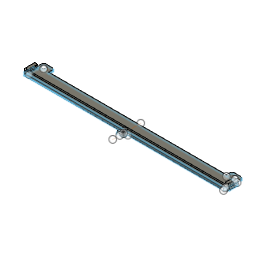
Light Bar v2 (Autodesk Fusion 360 design; units mm, degrees)
Autodesk Fusion 360 part; units mm, degrees
note: some values were not read from the file. Set by a fixed rule: which sketch regions a step uses.
sketch "base" plane through (0, 0, 0) normal (0, 1, 0) x (1, 0, 0)
  line L0 (-100, 1.5) -> (180, 1.5)
  line L1 (180, 1.5) -> (180, -13.5)
  line L2 (180, -13.5) -> (-100, -13.5)
  line L3 (-100, -13.5) -> (-100, 1.5)
  line L4 (-100, -13.5) -> (180, -13.5)
  line L5 (180, -13.5) -> (180, -17.5)
  line L6 (180, -17.5) -> (-100, -17.5)
  line L7 (-100, -17.5) -> (-100, -13.5)
  line L8 (-100, 1.5) -> (-85, 1.5) construction
  circle A0 centre (-94.5, 4) radius 2.5
  line L9 (-100, 1.5) -> (-100, 7.5)
  line L10 (-100, 7.5) -> (-98, 9.5)
  line L11 (-85, 1.5) -> (-85, 7.5)
  line L12 (-85, 7.5) -> (-87, 9.5)
  line L13 (-87, 9.5) -> (-98, 9.5)
  line L14 (40, 6.0385) -> (40, -33.3841) construction
  line L15 (167, 9.5) -> (178, 9.5)
  line L16 (180, 7.5) -> (178, 9.5)
  line L17 (180, 1.5) -> (180, 7.5)
  circle A1 centre (174.5, 4) radius 2.5
  line L18 (165, 7.5) -> (167, 9.5)
  line L19 (165, 1.5) -> (165, 7.5)
  circle A2 centre (40, -18.5) radius 2.5
  line L20 (34.5, -21.5) -> (36.5, -21.5) construction
  line L21 (36.5, -21.5) -> (36.5, -23.5) construction
  line L22 (34.5, -21.5) -> (36.5, -23.5)
  line L23 (36.5, -23.5) -> (40, -23.5)
  circle A3 centre (40, -18.5) radius 3.75 construction
  circle A4 centre (40, -18.5) radius 4
  line L24 (34.5, -21.5) -> (34.5, -17.5)
  line L25 (45.5, -21.5) -> (45.5, -17.5)
  line L26 (45.5, -21.5) -> (43.5, -23.5)
  line L27 (43.5, -23.5) -> (40, -23.5)
  line L28 (-98, -13) -> (-98, -1) construction
  line L29 (-98, -1) -> (-104, -1)
  line L30 (-104, -1) -> (-104, -13.5)
  line L31 (-104, -13.5) -> (-100, -17.5)
  line L32 (-98, -1) -> (-98, -13.5)
  line L33 (178, -13) -> (178, -1) construction
  line L34 (178, -1) -> (178, -13.5)
  line L35 (178, -1) -> (184, -1)
  line L36 (184, -1) -> (184, -13.5)
  line L37 (184, -13.5) -> (180, -17.5)
  circle A5 centre (-94.5, 4) radius 3.75 construction
  circle A6 centre (174.5, 4) radius 3.75 construction
  dimension "d1" = 280
  dimension "d2" = 15
  dimension "d3" = 4
  dimension "d4" = 280
  dimension "d5" = 15
  dimension "d7" = 5
  dimension "d8" = 2.5
  dimension "d11" = 140
  dimension "d16" = 5
  dimension "d17" = 5
  dimension "d20" = 2
  dimension "d21" = 2
  dimension "d22" = 7.5
  dimension "d23" = 8
  dimension "d29" = 12.5
  dimension "d42" = 7.5
  dimension "d43" = 7.5
  constraint horizontal L0
  constraint vertical L1
  constraint horizontal L2
  constraint vertical L3
  constraint horizontal L4
  constraint vertical L5
  constraint horizontal L6
  constraint vertical L7
  constraint horizontal L8
  constraint perpendicular L6 L14
  constraint symmetric L0.start L14 L0.end
  constraint symmetric L8.end L14 L19.start
  constraint symmetric A0 L14 A1
  constraint symmetric L9.end L14 L16.start
  constraint symmetric L10.end L14 L15.end
  constraint symmetric L11.end L14 L18.start
  constraint symmetric L12.end L14 L15.start
  constraint coincident L14 A2.centre
  constraint perpendicular L20 L21
  constraint coincident L14 L23.end
  constraint perpendicular L14 L23
  constraint concentric A2 A3
  constraint concentric A2 A4
  constraint coincident L6 L24.end
  constraint perpendicular L6 L24
  constraint symmetric L14 L20.start L25.start
  constraint symmetric L14 L21.end L26.end
  constraint symmetric L14 L23.end L27.end
  constraint symmetric L14 L24.end L25.end
  constraint parallel L3 L28
  constraint perpendicular L28 L29
  constraint perpendicular L29 L30
  constraint coincident L2 L32.end
  constraint perpendicular L2 L32
  constraint symmetric L6.end L14 L5.end
  constraint symmetric L14 L28.start L33.start
  constraint symmetric L14 L28.end L33.end
  constraint symmetric L14 L29.end L35.end
  constraint symmetric L14 L30.end L36.end
  constraint symmetric L14 L32.end L34.end
  constraint concentric A0 A5
  constraint concentric A1 A6
  measures "d1" distance of L0.start L0.end
  measures "d2" distance of L0.start L2.end
  measures "d3" distance of L2.end L6.end
  measures "d4" distance of L2.end L1.end
  measures "d5" distance of L0.start L8.end
  measures "d7" diameter of A0
  measures "d8" distance of L0 A0.centre
  measures "d11" distance of L3 L14
  measures "d16" diameter of A2
  measures "d17" distance of L4 A2.centre L0.start
  measures "d20" distance of L20.start L20.end L0.start
  measures "d21" distance of L20.end L21.end L0.start
  measures "d22" diameter of A3
  measures "d23" diameter of A4
  measures "d29" distance of L29.end L30.end
  measures "d42" diameter of A5
  measures "d43" diameter of A6
extrude "Extrude1" add sketch "base" along normal blind 2 contours L0 L1 L2 L3 L4 L29 L32 L34 L35 | L0 L9 L10 L11 L12 L13 | L0 L15 L16 L17 L18 L19 | L2 L3 L4 L29 L32 | L1 L2 L4 L34 L35 | L6 L22 L23 A4 L24 L25 L26 L27 | L6 A2 A4 | L6 A2 A4 makes body 1 at (-1.6667, 0, 8.5) makes body 2 at (39.9377, 0, 22.6643)
extrude "Extrude2" add sketch "base" along normal blind 5 contours L2 L4 L5 L6 L7 A4 bodies 1 2
chamfer "Chamfer1" distance 2 angle 45 2 edges at (-31.9365, 5, 17.5) (111.9365, 5, 17.5) on bodies 1
extrude "Extrude3" add sketch "base" along normal blind 6.5 contours L2 L3 L4 L29 L32 | L3 L7 L29 L30 L31 | L1 L5 L35 L36 L37 | L1 L2 L4 L34 L35 bodies 1
chamfer "Chamfer2" distance 2 angle 45 4 edges at (182, 6.5, 15.5) (184, 6.5, 7.25) (-102, 6.5, 15.5) (-104, 6.5, 7.25) on bodies 1
sketch "Sketch2" plane through (-104, 0, 0) normal (-1, 0, 0) x (0, 0, 1)
  line L0 (13.5, 4.5) -> (1, 4.5)
  line L1 (1, 4.5) -> (1, 0)
  line L2 (1, 0) -> (13.5, 0)
  line L3 (13.5, 0) -> (13.5, 4.5)
  circle A0 centre (3.2461, 4.25) radius 1.25
  line L4 (-7.5, 2) -> (1, 2)
  circle A1 centre (3.2461, 4.25) radius 1.25
  circle A2 centre (6.7461, 4.25) radius 1.25
  circle A3 centre (10.2461, 4.25) radius 1.25
  dimension "d33" = 2.5
  dimension "d36" = 2.25
  dimension "d37" = 2.5
  dimension "d38" = 2.5
  dimension "d39" = 2.5
  measures "d33" diameter of A0
  measures "d36" distance of A0.centre L4
  measures "d37" diameter of A1
  measures "d38" diameter of A2
  measures "d39" diameter of A3
extrude "Extrude4" cut sketch "Sketch2" against normal blind 300 contours L0 A3 | L0 A3 | L0 A2 | L0 A2 | L0 A0 A1 | L0 A0 A1 bodies 1
chamfer "Chamfer4" distance 2 angle 45 2 edges at (180, 5.75, 13.5) (-100, 5.75, 13.5) on bodies 1
